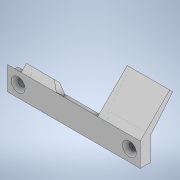
# Autodesk Inventor part: display_mount
Saved by Autodesk Inventor 2021 (Build 250183000, 183)
## iProperties
Created: 2024-09-18
Part Number: display_mount
Material: Generic
Document SubType Name: Modeling
Designer: Toby
Density: 1 g/cm^3
Appearance: Default
Author: Toby
Autodesk Inventor part; units mm, degrees
ref_plane "YZ Plane" through (0, 0, 0) normal (1, 0, 0) x (0, 1, 0)
ref_plane "XZ Plane" through (0, 0, 0) normal (0, 1, 0) x (-1, 0, 0)
ref_plane "XY Plane" through (0, 0, 0) normal (0, 0, 1) x (1, 0, 0)
sketch "Sketch1" plane through (0, 0, 0) normal (0, 0, 1) x (1, 0, 0)
  line L0 (-19.1, 3.4) -> (19.1, 3.4)
  line L1 (19.1, 3.4) -> (19.1, -3.4)
  line L2 (19.1, -3.4) -> (-19.1, -3.4)
  line L3 (-19.1, -3.4) -> (-19.1, 3.4)
  point P0 (0, 0)
  dimension "d0" = 38.2
  dimension "d1" = 6.8
  dimension "d2" = 19.1
  dimension "d3" = 3.4
  constraints: 8 end point, 2 parallel, 1 horizontal, 1 perpendicular
  measures "d0" distance of L0.start L0.end
  measures "d1" distance of L2.end L0.start
  measures "d2" distance from line of point (0, 0) L3
  measures "d3" distance from line of point (0, 0) L0
extrude "Extrusion1" add sketch "Sketch1" along normal blind 3
sketch "Sketch2" plane through (0, 0, 3) normal (0, 0, 1) x (1, 0, 0)
  line L0 (19.1, 3.4) -> (-19.1, 3.4) projected
  line L1 (-19.1, 3.4) -> (-19.1, -3.4) projected
  line L2 (19.1, -3.4) -> (19.1, 3.4) projected
  point P0 (0, 0)
  point P1 (-16, -0.1)
  point P2 (16, -0.1)
  point P3 (-16, -0.1)
  dimension "d6" = 3.5
  dimension "d7" = 3.5
  dimension "d8" = 32
  dimension "d9" = 3.1
  dimension "d10" = 3.1
  constraints: 1 coincident
  measures "d6" distance from line of point (-16, -0.1) L0
  measures "d7" distance from line of L0 point (16, -0.1)
  measures "d8" distance of point (16, -0.1) point (-16, -0.1)
  measures "d9" distance from line of L1 point (-16, -0.1)
  measures "d10" distance from line of L2 point (16, -0.1)
hole "Hole1" at (-16, -0.1, 3) at (16, -0.1, 3) direction (0, 0, -1) diameter 2 depth 4 tip angle 118 countersink diameter 4 countersink angle 90
sketch "Sketch3" plane through (19.1, -3.4, 0) normal (1, 0, 0) x (0, 0, -1)
  line L0 (-3, 6.8) -> (-3, 0) projected
  line L1 (-3, 6.8) -> (5.4853, 15.2853)
  line L2 (-3, 6.8) -> (9, 6.8) construction
  line L3 (5.4853, 15.2853) -> (6.3338, 14.4368)
  line L4 (0, 0) -> (0, 6.8) projected
  line L5 (6.3338, 14.4368) -> (0, 6.8)
  line L6 (0, 6.8) -> (-3, 6.8)
  point P0 (0, 3.4)
  dimension "d18" = 12
  dimension "d19" = 45
  dimension "d20" = 1.2
  constraints: 10 end point, 2 perpendicular, 1 equal length, 1 horizontal
  measures "d18" distance of L0.start L1.end
  measures "d19" angle of L2 L1
  measures "d20" distance of L1.end L3.end
extrude "Extrusion2" add sketch "Sketch3" against normal blind 38.2
sketch "Sketch4" plane through (-19.1, 11.8853, -5.4853) normal (0, 0.7071, 0.7071) x (1, 0, 0)
  line L0 (0, -12) -> (0, 0) projected
  line L1 (38.2, -12) -> (0, -12) projected
  line L2 (0, 0) -> (4, 0)
  line L3 (4, 0) -> (4, -12)
  line L4 (4, -12) -> (0, -12)
  line L5 (0, -12) -> (0, 0)
  line L6 (38.2, 0) -> (0, 0) projected
  line L7 (38.2, -9.8787) -> (0, -9.8787) projected
  line L8 (4, 0) -> (14, 0)
  line L9 (14, 0) -> (14, -9.8787)
  line L10 (14, -9.8787) -> (4, -9.8787)
  line L11 (4, -9.8787) -> (4, 0)
  line L12 (14, 0) -> (26, 0)
  line L13 (26, 0) -> (26, -12)
  line L14 (26, -12) -> (14, -12)
  line L15 (14, -12) -> (14, 0)
  point P0 (19.1, -12.2828)
  point P1 (4, -9.8787)
  point P2 (14, -9.8787)
  dimension "d23" = 4
  dimension "d24" = 4
  dimension "d25" = 14
  dimension "d26" = 26
  constraints: 24 end point, 6 parallel, 4 point on line, 3 horizontal, 3 perpendicular
  measures "d23" distance between parallel lines of L0 L3
  measures "d24" distance between parallel lines of L0 L11
  measures "d25" distance between parallel lines of L0 L15
  measures "d26" distance between parallel lines of L0 L13
extrude "Extrusion3" cut sketch "Sketch4" against normal blind 3 contours L0 L7 L3 L1 | L0 L2 L3 L7 | L3 L6 L9 L7 | L15 L7 L13 L1 | L9 L6 L13 L7
sketch "Sketch5" plane through (0, 0, 0) normal (0, 0, -1) x (-1, 0, 0)
  line L0 (5.1, 2.1574) -> (-6.9, 2.1574) projected
  line L1 (-6.9, 1.2787) -> (5.1, 1.2787) projected
  line L2 (-6.9, 2.1574) -> (5.1, 2.1574)
  line L3 (5.1, 2.1574) -> (5.1, 1.2787)
  line L4 (5.1, 1.2787) -> (-6.9, 1.2787)
  line L5 (-6.9, 1.2787) -> (-6.9, 2.1574)
  line L6 (15.1, 2.1574) -> (15.1, 1.2787) projected
  line L7 (15.1, 1.2787) -> (19.1, 1.2787) projected
  line L8 (15.1, 2.1574) -> (19.1, 2.1574)
  line L9 (19.1, 2.1574) -> (19.1, 1.2787)
  line L10 (19.1, 1.2787) -> (15.1, 1.2787)
  line L11 (15.1, 1.2787) -> (15.1, 2.1574)
  point P0 (0, 0)
  constraints: 16 end point, 4 parallel, 2 horizontal, 2 perpendicular
extrude "Extrusion4" cut sketch "Sketch5" against normal blind 0.88
chamfer "Chamfer1" distance 2 angle 45 1 edges at (-5.1, 4.15, 0.75)
body "Solid1"
